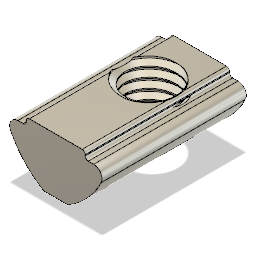
2020 Drop-in T-nut, M5 v4 (Autodesk Fusion 360 design; units mm, degrees)
Autodesk Fusion 360 part; units mm, degrees
sketch "Sketch1" plane through (0, 0, 0) normal (0, 0, 1) x (1, 0, 0)
  line L0 (0, 0) -> (0, -7.1858) construction
  line L1 (0, 0) -> (2.2, 0)
  line L2 (2.45, -0.25) -> (2.45, -0.35)
  line L3 (2.7, -0.6) -> (3.15, -0.6)
  arc A0 (3.7797, -1.6058) -> (3.15, -0.6) centre (3.15, -1.3) ccw
  line L4 (1, -4.6) -> (0, -4.6)
  arc A1 (1, -4.6) -> (3.7797, -1.6058) centre (-2.517, 1.4523) ccw
  arc A2 (2.45, -0.25) -> (2.2, 0) centre (2.2, -0.25) ccw
  arc A3 (2.45, -0.35) -> (2.7, -0.6) centre (2.7, -0.35) ccw
  line L5 (-2.45, -0.25) -> (-2.45, -0.35)
  line L6 (0, 0) -> (-2.2, 0)
  line L7 (-2.7, -0.6) -> (-3.15, -0.6)
  arc A4 (-2.7, -0.6) -> (-2.45, -0.35) centre (-2.7, -0.35) ccw
  arc A5 (-2.2, 0) -> (-2.45, -0.25) centre (-2.2, -0.25) ccw
  arc A6 (-3.7797, -1.6058) -> (-1, -4.6) centre (2.517, 1.4523) ccw
  line L8 (-1, -4.6) -> (0, -4.6)
  arc A7 (-3.15, -0.6) -> (-3.7797, -1.6058) centre (-3.15, -1.3) ccw
  dimension "d1" = 4.6
  dimension "d2" = 0.6
  dimension "d3" = 3.85
  dimension "d4" = 2.45
  dimension "d5" = 0.7
  dimension "d7" = 1
  dimension "d8" = 7
  dimension "d9" = 0.25
  dimension "d10" = 0.25
  constraint coincident L0.start L1.start
  constraint vertical L0
  constraint perpendicular L0 L1
  constraint perpendicular L1 L2
  constraint perpendicular L2 L3
  constraint tangent L3 A0
  constraint coincident L0 L4.end
  constraint perpendicular L0 L4
  constraint tangent A0 A1
  constraint tangent L1 A2
  constraint tangent L2 A2
  constraint tangent L2 A3
  constraint tangent L3 A3
  constraint symmetric L1.start L0 L6.start
  constraint symmetric L0 L1.start L6.start
  constraint symmetric L0 L3.end L7.end
  constraint symmetric L0 A0.start A6.start
  constraint symmetric L0 A0 A7
  constraint symmetric L0 L4.start A6.end
  constraint symmetric L0 L4.end L8.end
  constraint symmetric L0 A1 A6
  constraint symmetric L0 L1.end L6.end
  constraint symmetric L0 L2.start L5.start
  constraint symmetric L0 A2 A5
  constraint symmetric L0 L2.end L5.end
  constraint symmetric L0 L3.start L7.start
  constraint symmetric L0 A3 A4
  measures "d1" distance of L1 L4
  measures "d2" distance of L1 L3
  measures "d4" distance of L0 L2
  measures "d5" radius of A0
  measures "d7" distance of L4.start L4.end
  measures "d8" radius of A1
  measures "d9" radius of A2
  measures "d10" radius of A3
extrude "Extrude1" add sketch "Sketch1" against normal blind 12 makes body 1
sketch "Sketch2" plane through (0, 0, 0) normal (0, 1, 0) x (-1, 0, 0)
  line L0 (2.2, 0) -> (-2.2, 0)
  line L1 (-2.2, 0) -> (-2.2, -12)
  line L2 (-2.2, -12) -> (2.2, -12)
  line L3 (2.2, -12) -> (2.2, 0)
  point P0 (0, -8)
  point P1 (0, -3)
  dimension "d13" = 8
  dimension "d14" = 3
  constraint vertical origin P0
  constraint vertical origin P1
  measures "d13" distance of L0 P0
  measures "d14" distance of L0 P1
hole "Hole1" at (0, 0, -8) direction (0, -1, 0) diameter 4.234 end through all bodies 1
thread "Thread1" "ISO Metric profile 5.0 M5x0.8 6H" major diameter 5.12 minor diameter 4.234 pitch 0.8 angle 60 modelled right hand crest width 0.1 on face at (0.155, -1.5333, -10.1113) crest through (0, 0.45, -5.883) on bodies 1
sketch "Sketch3" plane through (0, 0, 0) normal (1, 0, 0) x (0, 0, -1)
  line L0 (0, -4.6) -> (5.8544, -4.6)
  line L1 (0, -1.6058) -> (0, -4.6)
  line L2 (4.5, -4.1) -> (1.5, -4.1)
  arc A0 (1.5, -4.1) -> (4.5, -4.1) centre (3, -4.1) ccw
  dimension "d18" = 3
  dimension "d19" = 1
  dimension "d20" = 3
  constraint horizontal L2
  constraint coincident A0.centre L2
  measures "d18" diameter of A0
  measures "d19" distance of L0 A0
  measures "d20" distance of A0.centre L1
revolve "Revolve1" cut sketch "Sketch3" angle 360 about axis through (0, -4.1, -4.5) along (0, 0, 1) bodies 1
sphere "SpherePrimitive1" add diameter 3 placed x (0, 0, -1) y (0, 1, 0) z (1, 0, 0) at (0, -7.0901, -5.4567) separate body makes body 2
move_body "Move1" bodies 2 to x (1, 0, 0) y (0, 1, 0) z (0, 0, 1) at (0, 3.208, 2.4505)
equation "d3 = ( 7.7 / 2 ) * 1 mm"
equation "d4 = ( 4.9 / 2 ) * 1 mm"
